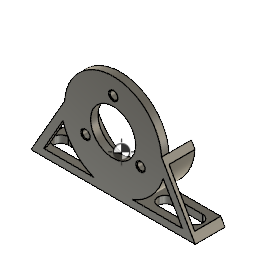
mount (Autodesk Fusion 360 design; units mm, degrees)
Autodesk Fusion 360 part; units mm, degrees
sketch "Skizze1" plane through (0, 0, 0) normal (0, 1, 0) x (1, 0, 0)
  line L0 (0, 0) -> (0, -13)
  line L1 (0, 0) -> (13, 0)
  arc A0 (0, -13) -> (13, 0) centre (0, 0) ccw
  dimension "d1" = 13
  dimension "d2" = 13
  constraint coincident L0.start L1.start
  constraint vertical L0
  constraint perpendicular L0 L1
  measures "d1" distance of L0.start L0.end
  measures "d2" distance of L0.start L1.end
extrude "Extrusion1" add sketch "Skizze1" along normal blind 2
revolve "Drehen1" add 1 faces at (0, 1.3333, 4.3333) angle 360 about axis through (0, 1.75, 0) along (0, 1, 0)
sketch "Skizze2" plane through (0, 0, 0) normal (0, -1, 0) x (1, 0, 0)
  circle A0 centre (0, 0) radius 13
  line L0 (0, 0) -> (0, 6)
  line L1 (0, 0) -> (6, 0)
  arc A1 (6, 0) -> (0, 6) centre (0, 0) ccw
  dimension "d6" = 6
  dimension "d7" = 6
  constraint coincident A0.centre L0.start
  constraint vertical L0
  constraint perpendicular L0 L1
  measures "d6" distance of A0.centre L0.end
  measures "d7" distance of A0.centre L1.end
extrude "Extrusion2" cut sketch "Skizze2" against normal blind 2 contours L0 L1 A1
revolve "Drehen2" cut 1 faces at (0, 0.6667, 2) angle 360 about axis through (0, 1.75, 0) along (0, 1, 0)
sketch "Skizze3" plane through (0, 0, 0) normal (0, -1, 0) x (1, 0, 0)
  circle A0 centre (0, 0) radius 6
  circle A1 centre (0, 0) radius 13
  circle A2 centre (0, 0) radius 8.5
  point P0 (0.0417, 8.4999)
  point P1 (-7.382, -4.2138)
  point P2 (7.3403, -4.2861)
  dimension "d11" = 17
  dimension "d12" = 120
  dimension "d13" = 120
  constraint coincident A0.centre A1.centre
  constraint coincident A2 P0
  constraint coincident A2 P1
  constraint coincident A2 P2
  measures "d11" diameter of A2
  measures "d12" angle of A0.centre P1 P2
  measures "d13" angle of A0.centre P0 P1
hole "Bohrung1" at (0.0417, 0, 8.4999) at (7.3403, 0, -4.2861) at (-7.382, 0, -4.2138) direction (0, 1, 0) diameter 2.1 depth 2 tip angle 180 countersink diameter 2.5 countersink angle 90
sketch "Skizze4" plane through (0, 0, 0) normal (0, -1, 0) x (1, 0, 0)
  circle A0 centre (7.3403, -4.2861) radius 1.25
  circle A1 centre (0.0417, 8.4999) radius 1.25
  circle A2 centre (-7.382, -4.2138) radius 1.25
  circle A3 centre (0, 0) radius 6
  circle A4 centre (0, 0) radius 13
  line L0 (0, -15) -> (-22, -15)
  line L1 (0, -15) -> (22, -15)
  line L2 (-22, -15) -> (-12.9777, 0.7613)
  line L3 (22, -15) -> (12.9777, 0.7613)
  dimension "d19" = 22
  dimension "d20" = 22
  dimension "d21" = 15
  constraint horizontal L0
  constraint parallel L0 L1
  constraint coincident A4 L2.end
  constraint coincident A4 L3.end
  measures "d19" distance of L0.start L0.end
  measures "d20" distance of L0.start L1.end
  measures "d21" distance of A3.centre L0.start
extrude "Extrusion3" add sketch "Skizze4" against normal blind 2 contours A4 L0 L1 L2 L3
sketch "Skizze5" plane through (0, 2, 0) normal (0, 1, 0) x (-1, 0, 0)
  circle A0 centre (-7.3403, -4.2861) radius 1.05
  circle A1 centre (-0.0417, 8.4999) radius 1.05
  circle A2 centre (7.382, -4.2138) radius 1.05
  arc A3 (12.9777, 0.7613) -> (-12.9777, 0.7613) centre (0, 0) ccw
  line L0 (-12.9777, 0.7613) -> (-22, -15)
  line L1 (-22, -15) -> (22, -15)
  line L2 (22, -15) -> (12.9777, 0.7613)
  circle A4 centre (0, 0) radius 6
  arc A5 (-12.9777, 0.7613) -> (12.9777, 0.7613) centre (0, 0) ccw
  arc A6 (-13.9666, -0.9663) -> (13.9666, -0.9663) centre (0, 0) ccw
  line L3 (-13.9666, -0.9663) -> (-12.9777, 0.7613)
  line L4 (13.9666, -0.9663) -> (12.9777, 0.7613)
  point P0 (-13.9666, -0.9663)
  point P1 (13.9666, -0.9663)
  dimension "d25" = 1
  constraint coincident A3.start L2.end
  constraint coincident A3.end L0.start
  constraint coincident A3.centre A4.centre
  constraint coincident L0 P0
  constraint coincident L2 P1
  constraint coincident P1 A6.end
  constraint coincident P0 A6.start
  measures "d25" distance of A5 A6
extrude "Extrusion4" add sketch "Skizze5" along normal blind 2 contours L0 L2 A5 A6 L3 L4
sketch "Skizze6" plane through (0, 2, 0) normal (0, 1, 0) x (-1, 0, 0)
  arc A0 (-13.9666, -0.9663) -> (13.9666, -0.9663) centre (0, 0) ccw
  line L0 (-13.9666, -0.9663) -> (-22, -15)
  line L1 (-22, -15) -> (22, -15)
  line L2 (22, -15) -> (13.9666, -0.9663)
  line L3 (-22, -15) -> (22, -15)
  line L4 (-22, -15) -> (-20.8551, -13)
  line L5 (-20.8551, -13) -> (20.8551, -13)
  line L6 (20.8551, -13) -> (22, -15)
  dimension "d28" = 2
  constraint coincident L0.end L1.start
  constraint coincident L1.end L2.start
  constraint coincident L0 L4.end
  constraint parallel L0 L4
  constraint coincident L2 L5.end
  constraint parallel L3 L5
  measures "d28" distance of L3 L5
extrude "Extrusion5" add sketch "Skizze6" along normal blind 6 contours A0 L0 L1 L2 L3 L4 L5 L6
extrude "Extrusion6" add 1 faces at (6.6033, 4, -11.556) along direction (0, 1, 0) blind 4
sketch "Skizze8" plane through (0, 2, 0) normal (0, 1, 0) x (-1, 0, 0)
  line L0 (-20.8551, -13) -> (-5.1962, -13)
  arc A0 (-13.9666, -0.9663) -> (-5.1962, -13) centre (0, 0) ccw
  line L1 (-13.9666, -0.9663) -> (-20.8551, -13)
  line L2 (-13.4103, -4.0203) -> (-18.5506, -13)
  line L3 (-18.5506, -13) -> (-5.1962, -13)
  dimension "d42" = 2
  constraint coincident A0 L2.start
  constraint coincident L0 L2.end
  constraint parallel L1 L2
  constraint coincident L0.end A0.end
  measures "d42" distance of L1 L2
extrude "Extrusion7" cut sketch "Skizze8" against normal blind 2 contours L0 A0 L2 L3
sketch "Skizze9" plane through (0, 2, 0) normal (0, 1, 0) x (-1, 0, 0)
  line L0 (5.1962, -13) -> (20.8551, -13)
  line L1 (20.8551, -13) -> (13.9666, -0.9663)
  arc A0 (5.1962, -13) -> (13.9666, -0.9663) centre (0, 0) ccw
  line L2 (13.4103, -4.0203) -> (18.5506, -13)
  dimension "d45" = 2
  constraint coincident A0 L2.start
  constraint coincident L0 L2.end
  constraint parallel L1 L2
  measures "d45" distance of L1 L2
extrude "Extrusion8" cut sketch "Skizze9" against normal blind 2 contours L0 A0 L2
extrude "Extrusion12" cut 1 faces at (17.6054, 2, -10.0068) along direction (0, -1, 0) blind 1
extrude "Extrusion13" cut 1 faces at (-17.6054, 2, -10.0068) along direction (0, -1, 0) blind 1
sketch "Skizze11" plane through (0, 0, -13) normal (0, 0, 1) x (-1, 0, 0)
  line L0 (5.1962, 0) -> (5.1962, -8)
  line L1 (5.1962, -8) -> (20.8551, -8)
  line L2 (20.8551, -8) -> (20.8551, -1)
  line L3 (20.8551, -1) -> (18.5506, -1)
  line L4 (18.5506, -1) -> (18.5506, 0)
  line L5 (18.5506, 0) -> (5.1962, 0)
  line L6 (22, 0) -> (12.9777, 0)
  line L7 (22, 0) -> (22, -8)
  line L8 (18, -6) -> (10, -6)
  line L9 (18, -2) -> (10, -2)
  arc A0 (10, -2) -> (10, -6) centre (10, -4) ccw
  arc A1 (18, -6) -> (18, -2) centre (18, -4) ccw
  line L10 (0, -19) -> (0, 8)
  line L11 (-22, 0) -> (-22, -8)
  line L12 (-18, -2) -> (-10, -2)
  line L13 (-18, -6) -> (-10, -6)
  arc A2 (-18, -2) -> (-18, -6) centre (-18, -4) ccw
  arc A3 (-10, -6) -> (-10, -2) centre (-10, -4) ccw
  point P0 (18, -6)
  point P1 (10, -6)
  point P2 (10, -2)
  point P3 (18, -2)
  point P4 (18, -4)
  point P5 (10, -4)
  dimension "d80" = 2
  dimension "d81" = 2
  dimension "d82" = 2
  dimension "d83" = 2
  dimension "d84" = 4
  dimension "d86" = 4
  dimension "d87" = 8
  dimension "d88" = 8
  dimension "d89" = 2
  dimension "d90" = 2
  dimension "d91" = 4
  dimension "d92" = 8
  dimension "d93" = 22
  dimension "d94" = 22
  constraint coincident P0 L8.start
  constraint coincident P1 L8.end
  constraint coincident P3 L9.start
  constraint coincident P2 L9.end
  constraint coincident P5 A0.centre
  constraint coincident P4 A1.centre
  constraint vertical L10
  constraint symmetric P0 L10 L13.start
  constraint symmetric P1 L10 L13.end
  constraint symmetric P3 L10 L12.start
  constraint symmetric P2 L10 L12.end
  constraint symmetric A0 L10 A3
  constraint symmetric A1 L10 A2
  measures "d80" distance of L1 P0
  measures "d81" distance of P3 L6
  measures "d82" distance of L5 P2
  measures "d83" distance of L1 P1
  measures "d84" distance of P0 L7
  measures "d86" distance of P3 L7
  measures "d87" distance of P0 P1
  measures "d88" distance of P2 P3
  measures "d89" vertical distance of P0 P4
  measures "d90" vertical distance of P1 P5
  measures "d91" distance of L7 P4
  measures "d92" distance of P4 P5
  measures "d93" distance of L10 L11
  measures "d94" distance of L7 L10
extrude "Extrusion14" cut sketch "Skizze11" against normal blind 2 contours L8 L9 A0 A1 | L12 L13 A2 A3
